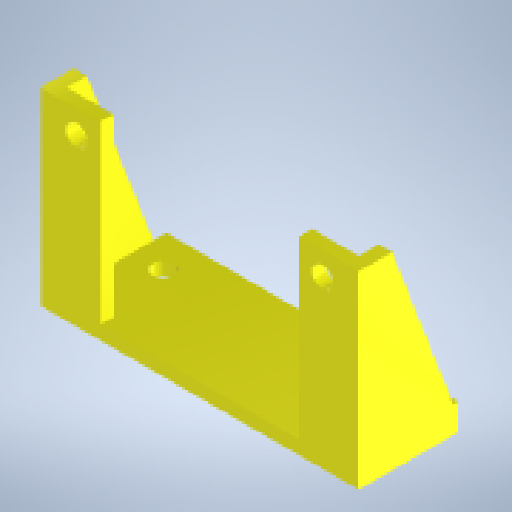
# Autodesk Inventor part: SPG27_Braket
Saved by Autodesk Inventor 2025.3 (Build 293356000, 356)
## iProperties
Created: 2025-08-17
Part Number: SPG27_Braket
Material: 一般
Document SubType Name: Modeling
Designer: daisuke
Density: 1 g/cm^3
Appearance: 滑らか - 黄
Author: daisuke
Autodesk Inventor part; units mm, degrees
ref_plane "YZ Plane" through (0, 0, 0) normal (1, 0, 0) x (0, 1, 0)
ref_plane "XZ Plane" through (0, 0, 0) normal (0, 1, 0) x (-1, 0, 0)
ref_plane "XY Plane" through (0, 0, 0) normal (0, 0, 1) x (1, 0, 0)
sketch "スケッチ1" plane through (0, 0, 0) normal (0, 0, 1) x (1, 0, 0)
  line L0 (-22, 0) -> (22, 0)
  line L1 (22, 0) -> (22, 17)
  line L2 (22, 17) -> (-22, 17)
  line L3 (-22, 17) -> (-22, 0)
  point P0 (0, 0)
  point P1 (0, 0)
  dimension "d0" = 44
  dimension "d1" = 17
  constraints: 8 end point, 2 parallel, 1 coincident, 1 horizontal, 1 midpoint, 1 perpendicular
  measures "d0" distance of L2.end L1.end
  measures "d1" distance of L1.end L0.end
extrude "土台" add sketch "スケッチ1" along normal blind 2
sketch "スケッチ2" plane through (-22, 0, 0) normal (0, -1, 0) x (1, 0, 0)
  line L0 (22, 0) -> (22, 53.3234) construction
  circle A0 centre (22, 25) radius 15 construction
  line L1 (0, 2) -> (44, 2) construction
  line L2 (-7.4711, 25) -> (51.4711, 25) construction
  circle A1 centre (3.5, 25) radius 1.6
  circle A2 centre (40.5, 25) radius 1.6
  line L3 (0, 2) -> (7, 2)
  line L4 (7, 2) -> (7, 28.5)
  line L5 (7, 28.5) -> (0, 28.5)
  line L6 (0, 28.5) -> (0, 2)
  line L7 (44, 2) -> (37, 2)
  line L8 (37, 2) -> (37, 28.5)
  line L9 (37, 28.5) -> (44, 28.5)
  line L10 (44, 28.5) -> (44, 2)
  dimension "d4" = 30
  dimension "d5" = 23
  dimension "d6" = 3.2
  dimension "d7" = 37
  dimension "d8" = 3.5
  constraints: 20 end point, 4 parallel, 4 point on line, 3 centre point, 3 horizontal, 2 perpendicular, 2 tangent, 1 equal radius, 1 midpoint, 1 symmetric about line, 1 vertical
  measures "d4" diameter of A0
  measures "d5" distance from line of A0.centre L1
  measures "d6" diameter of A1
  measures "d7" distance of A2.centre A1.centre
  measures "d8" distance between parallel lines of L2 L5
extrude "モータ支柱" add sketch "スケッチ2" against normal blind 2
sketch "スケッチ3" plane through (22, 0, 0) normal (1, 0, 0) x (0, 0, -1)
  line L0 (-28.5, 0) -> (-28.5, 2) projected
  line L1 (-28.5, 0) -> (-28.5, 5)
  line L2 (-28.5, 5) -> (-2, 15)
  line L3 (-2, 17) -> (-2, 2) projected
  line L4 (0, 17) -> (0, 0) projected
  line L5 (0, 15) -> (-2, 15)
  line L6 (0, 0) -> (-28.5, 0) projected
  dimension "d11" = 5
  dimension "d12" = 15
  constraints: 6 end point, 2 point on line, 1 perpendicular, 1 vertical
  measures "d11" distance of L0.start L1.end
  measures "d12" distance between parallel lines of L6 L5
extrude "補強リブ" add sketch "スケッチ3" along normal blind 2
mirror "ミラー1" about plane through (0, 0, 0) normal (1, 0, 0) of "補強リブ"
sketch "スケッチ4" plane through (0, 0, 2) normal (0, 0, 1) x (1, 0, 0)
  line L0 (0, 0) -> (0, 42.8792) construction
  line L1 (-15, 0) -> (15, 0) construction
  line L2 (22, 17) -> (-22, 17) projected
  point P0 (-17.5, 13)
  point P1 (17.5, 13)
  point P2 (0, 0)
  dimension "d15" = 35
  dimension "d24" = 4
  constraints: 2 end point, 1 midpoint, 1 symmetric about line, 1 vertical
  measures "d15" distance of point (17.5, 13) point (-17.5, 13)
  measures "d24" distance from line of L2 point (17.5, 13)
hole "穴1" at (-17.5, 13, 2) at (17.5, 13, 2) direction (0, 0, -1) diameter 3.2 end through all
